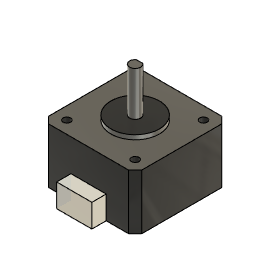
Nema17_25mm v1 v1 (Autodesk Fusion 360 design; units mm, degrees)
Autodesk Fusion 360 part; units mm, degrees
note: some values were not read from the file. Set by a fixed rule: which sketch regions a step uses.
sketch "Esquisse1" plane through (0, 0, 0) normal (0, 0, 1) x (1, 0, 0)
  line L0 (21.15, 21.15) -> (-21.15, 21.15)
  line L1 (-21.15, 21.15) -> (-21.15, -21.15)
  line L2 (-21.15, -21.15) -> (21.15, -21.15)
  line L3 (21.15, -21.15) -> (21.15, 21.15)
  line L4 (21.15, 21.15) -> (-21.15, -21.15) construction
  line L5 (-21.15, 21.15) -> (21.15, -21.15) construction
  dimension "d1" = 42.3
  dimension "d2" = 42.3
  constraint horizontal L0
  constraint perpendicular L0 L1
  constraint parallel L0 L2
  constraint parallel L1 L3
  constraint coincident L4 origin
  constraint coincident L5 origin
  measures "d1" distance of L1.end L2.end
  measures "d2" distance of L0.end L1.end
extrude "Extrusion1" add sketch "Esquisse1" along normal blind 25
sketch "Esquisse2" plane through (0, 0, 25) normal (0, 0, 1) x (-1, 0, 0)
  line L0 (-21.15, 21.15) -> (-21.15, -21.15)
  line L1 (-21.15, -21.15) -> (21.15, -21.15)
  line L2 (21.15, -21.15) -> (21.15, 21.15)
  line L3 (21.15, 21.15) -> (-21.15, 21.15)
  circle A0 centre (15.5, -15.5) radius 1.7
  circle A1 centre (-15.5, -15.5) radius 1.7
  circle A2 centre (15.5, 15.5) radius 1.7
  circle A3 centre (-15.5, 15.5) radius 1.7
  dimension "d5" = 3.4
  dimension "d6" = 3.4
  dimension "d7" = 3.4
  dimension "d8" = 3.4
  dimension "d9" = 5.65
  dimension "d10" = 5.65
  dimension "d11" = 5.65
  dimension "d12" = 5.65
  dimension "d13" = 5.65
  dimension "d14" = 5.65
  dimension "d15" = 5.65
  dimension "d16" = 5.65
  measures "d5" diameter of A0
  measures "d6" diameter of A1
  measures "d7" diameter of A3
  measures "d8" diameter of A2
  measures "d9" distance of L2 A0.centre
  measures "d10" distance of L1 A0.centre
  measures "d11" distance of L1 A1.centre
  measures "d12" distance of L0 A1.centre
  measures "d13" distance of L2 A2.centre
  measures "d14" distance of L3 A2.centre
  measures "d15" distance of L0 A3.centre
  measures "d16" distance of L3 A3.centre
extrude "Extrusion2" cut sketch "Esquisse2" against normal blind 13.5 contours A0 | A1 | A2 | A3
sketch "Esquisse3" plane through (0, 0, 25) normal (0, 0, 1) x (-1, 0, 0)
  circle A0 centre (-15.5, -15.5) radius 1.7
  circle A1 centre (-15.5, 15.5) radius 1.7
  circle A2 centre (15.5, -15.5) radius 1.7
  circle A3 centre (15.5, 15.5) radius 1.7
  line L0 (-21.15, 21.15) -> (-21.15, -21.15)
  line L1 (-21.15, -21.15) -> (21.15, -21.15)
  line L2 (21.15, -21.15) -> (21.15, 21.15)
  line L3 (21.15, 21.15) -> (-21.15, 21.15)
  circle A4 centre (0, 0) radius 11
  circle A5 centre (0, 0) radius 2.5
  dimension "d19" = 22
  dimension "d20" = 5
  constraint coincident A4.centre A5.centre
  constraint concentric A4 A5
  measures "d19" diameter of A4
  measures "d20" diameter of A5
extrude "Extrusion3" add sketch "Esquisse3" along normal blind 22 contours A5
extrude "Extrusion4" add sketch "Esquisse3" along normal blind 2 contours A4
sketch "Esquisse4" plane through (0, 0, 47) normal (0, 0, 1) x (-1, 0, 0)
  circle A0 centre (0, 0) radius 2.5
  line L0 (1.5, -2) -> (-1.5, -2)
  circle A1 centre (0, 0) radius 2.5
  dimension "d25" = 2
  constraint coincident A0 L0.start
  constraint coincident A0 L0.end
  constraint horizontal L0
  measures "d25" distance of L0 A0.centre
extrude "Extrusion5" cut sketch "Esquisse4" against normal blind 15 contours A0 L0 A1 picked at (-0.3999, -2.0645)
sketch "Esquisse5" plane through (0, 0, 0) normal (0, 0, -1) x (1, 0, 0)
  line L0 (21.15, -21.15) -> (21.15, 21.15)
  line L1 (21.15, 21.15) -> (-21.15, 21.15)
  line L2 (-21.15, 21.15) -> (-21.15, -21.15)
  line L3 (-21.15, -21.15) -> (21.15, -21.15)
  line L4 (8, 21.15) -> (-8, 21.15)
  line L5 (-8, 21.15) -> (-8, 27.65)
  line L6 (-8, 27.65) -> (8, 27.65)
  line L7 (8, 27.65) -> (8, 21.15)
  line L8 (8, 21.15) -> (-8, 27.65) construction
  line L9 (-8, 21.15) -> (8, 27.65) construction
  point P0 (0, 24.4)
  dimension "d28" = 6.5
  dimension "d29" = 16
  dimension "d30" = 13.15
  constraint horizontal L4
  constraint perpendicular L4 L5
  constraint parallel L4 L6
  constraint parallel L5 L7
  constraint coincident L1 L4.start
  constraint coincident L8 P0
  constraint coincident L9 P0
  measures "d28" distance of L4.start L6.end
  measures "d29" distance of L5.end L6.end
  measures "d30" distance of L0 L7
extrude "Extrusion6" add sketch "Esquisse5" against normal blind 10.5 contours L1 L4 L5 L6 L7
chamfer "Chanfrein1" distance 3 angle 45 4 edges at (21.15, 21.15, 12.5) (21.15, -21.15, 12.5) (-21.15, 21.15, 12.5) (-21.15, -21.15, 12.5)
